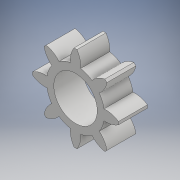
# Autodesk Inventor part: mtv_gear8_1-13
Saved by Autodesk Inventor 2018 (Build 220112000, 112)
## iProperties
Created: 2019-01-14
Part Number: mtv_gear8_1-13
Material: Generic
Document SubType Name: Modeling
Designer: aditya
Density: 1 g/cm^3
Appearance: Default
Author: aditya
## iProperties of the stored document mtv_gear8_1-13_3DPrint.ipt
Created: 2019-01-14
Part Number: mtv_gear8_1-13_3DPrint
Material: Generic
Document SubType Name: Modeling
Designer: aditya
Density: 1 g/cm^3
Appearance: Default
Author: aditya
Autodesk Inventor part; units mm, degrees
ref_plane "YZ Plane" through (0, 0, 0) normal (1, 0, 0) x (0, 1, 0)
ref_plane "XZ Plane" through (0, 0, 0) normal (0, 1, 0) x (-1, 0, 0)
ref_plane "XY Plane" through (0, 0, 0) normal (0, 0, 1) x (1, 0, 0)
sketch "Sketch1" plane through (0, 0, 0) normal (0, 1, 0) x (-1, 0, 0)
  circle A0 centre (0, 0) radius 1.5
  circle A1 centre (0, 0) radius 2
  dimension "d0" = 3
  dimension "d1" = 4
  constraints: 2 centre point, 2 coincident
  measures "d0" diameter of A0
  measures "d1" diameter of A1
extrude "Extrusion1" add sketch "Sketch1" along normal blind 2
sketch "Sketch2" plane through (0, 2, 0) normal (0, 1, 0) x (1, 0, 0)
  line L0 (-1.9117, -0.1) -> (-2.7237, -0.1) construction
  line L1 (-2.7237, -0.1) -> (-2.7237, 0.1) construction
  line L2 (-2.7237, 0.1) -> (-1.9117, 0.1) construction
  line L3 (-1.9117, 0.1) -> (-1.9117, -0.1) construction
  line L4 (-1.9117, 0) -> (-1.9117, 0.35) construction
  line L5 (-1.9117, 0) -> (-1.5617, 0) construction
  line L6 (-1.9117, 0.35) -> (-1.9117, -0.35) construction
  line L7 (-1.9117, 0.1) -> (-2.9669, 0.1) construction
  line L8 (-2.9669, 0.1) -> (-2.9669, -0.1) construction
  line L9 (-2.9669, -0.1) -> (-1.9117, -0.1) construction
  line L10 (-1.9117, -0.1) -> (-1.9117, 0.1) construction
  arc A0 (-2.9669, -0.1) -> (-1.9117, -0.35) centre (-2.1069, 1.1781) ccw construction
  arc A1 (-2.9669, -0.1) -> (-1.9117, -0.35) centre (-2.1069, 1.1781) ccw
  arc A2 (-1.9117, 0.35) -> (-2.9669, 0.1) centre (-2.1068, -1.1786) ccw
  line L11 (-2.9669, -0.1) -> (-2.9669, 0.1)
  line L12 (-1.9117, -0.35) -> (-1.9117, 0.35)
  point P0 (0, 0)
  dimension "d4" = 0.2
  dimension "d5" = 0.35
  dimension "d6" = 90
  dimension "d7" = 0.7
  dimension "d8" = 1.541
  constraints: 26 end point, 6 point on circle, 5 parallel, 3 centre point, 3 horizontal, 3 perpendicular, 1 collinear, 1 concentric, 1 midpoint, 1 point on line, 1 vertical
  measures "d4" distance of L0.end L1.end
  measures "d5" distance of L4.start L4.end
  measures "d6" angle of L5 L4
  measures "d7" distance of L4.end L6.end
  measures "d8" radius of A2
extrude "Extrusion2" add sketch "Sketch2" against normal blind 2
pattern_circular "Circular Pattern1" count 8 over 360 about axis through (0, 0, 0) along (0, 1, 0) of "Extrusion2"
body "Solid1"
